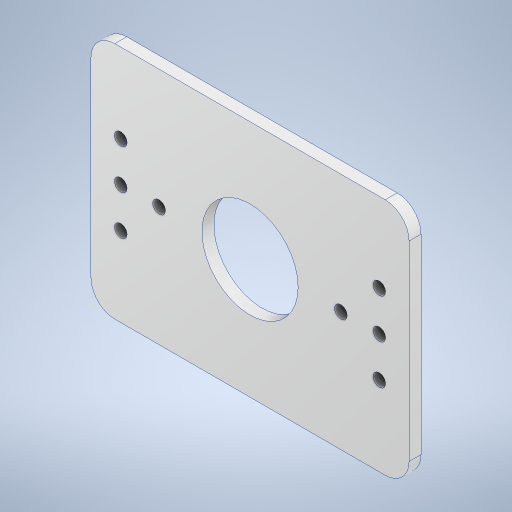
# Autodesk Inventor part: 射出_エンコーダー固定
Saved by Autodesk Inventor 2023 (Build 270158000, 158)
## iProperties
Created: 2022-04-20
Part Number: 射出_エンコーダー固定
Material: アルミニウム 6061
Document SubType Name: Modeling
Designer: yuta
Density: 2.7 g/cm^3
Appearance: アルミニウム - フラット
Author: yuta
Autodesk Inventor part; units mm, degrees
ref_plane "YZ Plane" through (0, 0, 0) normal (1, 0, 0) x (0, 1, 0)
ref_plane "XZ Plane" through (0, 0, 0) normal (0, 1, 0) x (-1, 0, 0)
ref_plane "XY Plane" through (0, 0, 0) normal (0, 0, 1) x (1, 0, 0)
sketch "スケッチ1" plane through (0, 0, 0) normal (0, 0, 1) x (1, 0, 0)
  line L0 (0, 0) -> (80, 0)
  line L1 (80, 0) -> (80, 60)
  line L2 (80, 60) -> (0, 60)
  line L3 (0, 60) -> (0, 0)
  dimension "d0" = 80
  dimension "d1" = 60
  constraints: 8 end point, 2 parallel, 1 horizontal, 1 perpendicular
  measures "d0" distance of L2.end L1.end
  measures "d1" distance of L1.end L0.end
extrude "押し出し1" add sketch "スケッチ1" along normal blind 3
sketch "スケッチ2" plane through (0, 0, 3) normal (0, 0, 1) x (1, 0, 0)
  point P0 (0, 0)
sketch "スケッチ3" plane through (0, 0, 3) normal (0, 0, 1) x (1, 0, 0)
  line L0 (0, 0) -> (80, 0) projected
  line L1 (15, 0) -> (15, 60) construction
  line L2 (15, 0) -> (75, 0) construction
  line L3 (0, 60) -> (0, 0) projected
  circle A0 centre (7.5, 30) radius 1.6
  circle A1 centre (7.5, 40) radius 1.6
  circle A2 centre (7.5, 20) radius 1.6
  line L4 (80, 60) -> (0, 60) projected
  line L5 (40, 60) -> (40, 0) construction
  circle A3 centre (72.5, 30) radius 1.6
  circle A4 centre (72.5, 40) radius 1.6
  circle A5 centre (72.5, 20) radius 1.6
  point P0 (0, 30)
  dimension "d4" = 60
  dimension "d5" = 90
  dimension "d6" = 15
  dimension "d7" = 3.2
  dimension "d8" = 7.5
  dimension "d9" = 30
  dimension "d10" = 3.2
  dimension "d11" = 3.2
  dimension "d12" = 10
  dimension "d13" = 10
  dimension "d14" = 40
  constraints: 6 centre point, 6 end point, 3 perpendicular, 3 symmetric about line, 2 midpoint, 2 point on line, 1 horizontal, 3 other
  measures "d4" distance of L1.start L1.end
  measures "d5" angle of L2 L1
  measures "d6" distance between parallel lines of L3 L1
  measures "d7" diameter of A0
  measures "d8" distance of point (0, 30) A0.centre
  measures "d9" distance from line of L0 A0.centre
  measures "d10" diameter of A1
  measures "d11" diameter of A2
  measures "d12" distance of A1.centre A0.centre
  measures "d13" distance of A2.centre A0.centre
  measures "d14" distance between parallel lines of L3 L5
hole "穴1" at (7.5, 40, 3) at (7.5, 30, 3) at (7.5, 20, 3) at (72.5, 40, 3) at (72.5, 30, 3) at (72.5, 20, 3) direction (0, 0, -1) diameter 3.2 end through all
sketch "スケッチ4" plane through (0, 0, 3) normal (0, 0, 1) x (1, 0, 0)
  circle A0 centre (40, 30) radius 7.5
  line L0 (80, 60) -> (0, 60) projected
  line L1 (80, 0) -> (80, 60) projected
  point P0 (0, 0)
  dimension "d22" = 15
  dimension "d23" = 30
  dimension "d24" = 40
  constraints: 1 centre point
  measures "d22" diameter of A0
  measures "d23" distance from line of L0 A0.centre
  measures "d24" distance from line of L1 A0.centre
extrude "押し出し2" cut sketch "スケッチ4" against normal blind 3
sketch "スケッチ5" plane through (0, 0, 3) normal (0, 0, 1) x (1, 0, 0)
  point P0 (0, 0)
sketch "スケッチ6" plane through (0, 0, 3) normal (0, 0, 1) x (1, 0, 0)
  circle A0 centre (40, 30) radius 7.5 projected
  circle A1 centre (40, 30) radius 12.1
  point P0 (0, 0)
  dimension "d27" = 24.2
  constraints: 1 centre point, 1 coincident
  measures "d27" diameter of A1
extrude "押し出し3" cut sketch "スケッチ6" against normal blind 3
sketch "スケッチ7" plane through (0, 0, 3) normal (0, 0, 1) x (1, 0, 0)
  circle A0 centre (40, 30) radius 12.1 projected
  line L0 (0, 0) -> (80, 0) projected
  point P0 (62.851, 30)
  point P1 (17.149, 30)
  dimension "d30" = 22.851
  dimension "d31" = 22.851
  dimension "d32" = 30
  dimension "d33" = 30
  measures "d30" distance of A0.centre point (62.851, 30)
  measures "d31" distance of point (17.149, 30) A0.centre
  measures "d32" distance from line of L0 point (17.149, 30)
  measures "d33" distance from line of L0 point (62.851, 30)
hole "穴2" at (17.149, 30, 3) at (62.851, 30, 3) direction (0, 0, -1) diameter 3.2 end through all
fillet "フィレット1" radius 6 4 edges at (0, 60, 1.5) (80, 60, 1.5) (80, 0, 1.5) (0, 0, 1.5)
sketch "スケッチ8" plane through (0, 0, 3) normal (0, 0, 1) x (1, 0, 0)
  point P0 (0, 0)
